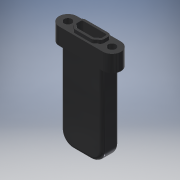
# Autodesk Inventor part: hdmi-panel-mount
Saved by Autodesk Inventor 2017 (Build 210142000, 142)
## iProperties
Created: 2020-10-05
Part Number: hdmi-panel-mount
Material: Generic
Document SubType Name: Modeling
Designer: Joe Ferner
Density: 1 g/cm^3
Appearance: Default
Author: Joe Ferner
Autodesk Inventor part; units mm, degrees
ref_plane "YZ Plane" through (0, 0, 0) normal (1, 0, 0) x (0, 1, 0)
ref_plane "XZ Plane" through (0, 0, 0) normal (0, 1, 0) x (-1, 0, 0)
ref_plane "XY Plane" through (0, 0, 0) normal (0, 0, 1) x (1, 0, 0)
sketch "Sketch1" plane through (0, 0, 0) normal (0, 0, 1) x (1, 0, 0)
  line L0 (0, 0) -> (26.3, 0)
  line L1 (26.3, 10.7) -> (0, 10.7)
  arc A0 (0, 10.7) -> (0, 0) centre (0, 5.35) ccw
  arc A1 (26.3, 0) -> (26.3, 10.7) centre (26.3, 5.35) ccw
  circle A2 centre (0, 5.35) radius 1.25
  circle A3 centre (26.3, 5.35) radius 1.25
  dimension "d0" = 26.3
  dimension "d1" = 10.7
  dimension "d2" = 2.5
  constraints: 4 centre point, 4 end point, 4 point on circle, 4 tangent, 2 coincident, 1 equal radius, 1 horizontal, 1 parallel
  measures "d0" distance of L0.start L0.end
  measures "d1" distance between parallel lines of L1 L0
  measures "d2" diameter of A2
extrude "Extrusion1" add sketch "Sketch1" against normal blind 10
sketch "Sketch2" plane through (0, 0, 0) normal (0, 0, 1) x (1, 0, 0)
  line L0 (0, 0) -> (26.3, 0) projected
  arc A0 (0, 10.7) -> (0, 0) centre (0, 5.35) ccw projected
  line L1 (6.9455, 3.7725) -> (7.7604, 2.8465)
  line L2 (8.361, 2.575) -> (17.939, 2.575)
  line L3 (18.5396, 2.8465) -> (19.3545, 3.7725)
  line L4 (19.6057, 3.9348) -> (20.0852, 4.0824)
  line L5 (20.65, 4.847) -> (20.65, 7.325)
  line L6 (19.85, 8.125) -> (6.45, 8.125)
  line L7 (5.65, 7.325) -> (5.65, 4.847)
  line L8 (6.2148, 4.0824) -> (6.6943, 3.9348)
  line L9 (26.3, 10.7) -> (0, 10.7) projected
  arc A1 (6.45, 8.125) -> (5.65, 7.325) centre (6.45, 7.325) ccw
  arc A2 (20.65, 7.325) -> (19.85, 8.125) centre (19.85, 7.325) ccw
  arc A3 (5.65, 4.847) -> (6.2148, 4.0824) centre (6.45, 4.847) ccw
  arc A4 (20.0852, 4.0824) -> (20.65, 4.847) centre (19.85, 4.847) ccw
  arc A5 (6.9455, 3.7725) -> (6.6943, 3.9348) centre (6.5326, 3.4092) ccw
  arc A6 (19.6057, 3.9348) -> (19.3545, 3.7725) centre (19.7674, 3.4092) ccw
  arc A7 (7.7604, 2.8465) -> (8.361, 2.575) centre (8.361, 3.375) ccw
  arc A8 (17.939, 2.575) -> (18.5396, 2.8465) centre (17.939, 3.375) ccw
  line L10 (6.45, 9.4895) -> (19.85, 9.4895)
  arc A9 (22.0145, 7.325) -> (19.85, 9.4895) centre (19.85, 7.325) ccw
  line L11 (22.0145, 7.325) -> (22.0145, 4.847)
  arc A10 (20.4865, 2.7782) -> (22.0145, 4.847) centre (19.85, 4.847) ccw
  line L12 (20.4865, 2.7782) -> (20.2268, 2.6983)
  line L13 (20.2268, 2.6983) -> (19.5639, 1.945)
  arc A11 (17.939, 1.2105) -> (19.5639, 1.945) centre (17.939, 3.375) ccw
  line L14 (17.939, 1.2105) -> (8.361, 1.2105)
  arc A12 (6.7361, 1.945) -> (8.361, 1.2105) centre (8.361, 3.375) ccw
  line L15 (6.7361, 1.945) -> (6.0732, 2.6983)
  line L16 (6.0732, 2.6983) -> (5.8135, 2.7782)
  arc A13 (4.2855, 4.847) -> (5.8135, 2.7782) centre (6.45, 4.847) ccw
  line L17 (4.2855, 4.847) -> (4.2855, 7.325)
  arc A14 (6.45, 9.4895) -> (4.2855, 7.325) centre (6.45, 7.325) ccw
  point P0 (6.8428, 3.8892)
  point P1 (7.9994, 2.575)
  point P2 (18.3006, 2.575)
  point P3 (19.4572, 3.8892)
  point P4 (20.65, 4.2561)
  point P5 (20.65, 8.125)
  point P6 (5.65, 8.125)
  point P7 (5.65, 4.2561)
  dimension "d25" = 15
  dimension "d26" = 5.55
  dimension "d27" = 5.65
  dimension "d28" = 2.575
  dimension "d29" = 0.8
  dimension "d30" = 0.8
  dimension "d32" = 107.1
  dimension "d34" = 107.1
  dimension "d35" = 41.35
  dimension "d36" = 41.35
  dimension "d37" = 0.55
  dimension "d38" = 0.8
  dimension "d39" = 2.711
  dimension "d40" = 2.711
  dimension "d42" = 2.478
  dimension "d43" = 2.478
  dimension "d44" = 1.3645
  constraints: 32 end point, 28 point on circle, 16 point on line, 16 tangent, 14 centre point, 4 equal radius, 4 parallel, 2 perpendicular, 13 other
  measures "d25" distance between parallel lines of L5 L7
  measures "d26" distance between parallel lines of L6 L2
  measures "d27" distance from line of A0.centre L7
  measures "d28" distance between parallel lines of L9 L6
  measures "d29" radius of A1
  measures "d30" radius of A3
  measures "d32" angle of L8 L7
  measures "d34" angle of L4 L5
  measures "d35" angle of L1 L7
  measures "d36" angle of L5 L3
  measures "d37" radius of A5
  measures "d38" radius of A7
  measures "d39" distance from line of L2.start L7
  measures "d40" distance from line of L2.end L5
  measures "d42" distance of L7.start L7.end
  measures "d43" distance of L5.start L5.end
  measures "d44" distance between parallel lines of L2 L14
extrude "Extrusion4" add sketch "Sketch2" along normal blind 2 contours A5 L8 A3 L7 A1 L6 A2 L5 A4 L4 A6 L3 A8 L2 A7 L1 | L10 A9 L11 A10 L12 L13 A11 L14 A12 L15 L16 A13 L17 A14
extrude "Extrusion5" cut sketch "Sketch2" against normal blind 4 and the other way blind 2 contours A5 L8 A3 L7 A1 L6 A2 L5 A4 L4 A6 L3 A8 L2 A7 L1
sketch "Sketch3" plane through (0, 0, -10) normal (0, 0, -1) x (-1, 0, 0)
  line L0 (-23.4, 0) -> (-2.9, 0)
  line L1 (-2.9, 0) -> (-2.9, 10.7)
  line L2 (-2.9, 10.7) -> (-23.4, 10.7)
  line L3 (-23.4, 10.7) -> (-23.4, 0)
  line L4 (0, 10.7) -> (-26.3, 10.7) projected
  arc A0 (-26.3, 10.7) -> (-26.3, 0) centre (-26.3, 5.35) ccw projected
  line L5 (-26.3, 0) -> (0, 0) projected
  dimension "d47" = 20.5
  dimension "d51" = 2.9
  constraints: 8 end point, 2 collinear, 2 parallel, 1 horizontal, 1 perpendicular
  measures "d47" distance of L0.start L0.end
  measures "d51" distance from line of A0.centre L3
extrude "Extrusion6" add sketch "Sketch3" along normal blind 24 contours L3 L2 L1 L0
sketch "Sketch4" plane through (2.9, 10.7, -10) normal (0, 1, 0) x (-1, 0, 0)
  line L0 (-20.5, 0) -> (-20.5, -24) projected
  line L1 (-20.5, -24) -> (0, -24) projected
  arc A0 (-20.5, -21) -> (-17.5, -24) centre (-17.5, -21) ccw
  arc A1 (-3, -24) -> (0, -21) centre (-3, -21) ccw
  line L2 (-20.5, -21) -> (-20.5, -24)
  line L3 (-20.5, -24) -> (-17.5, -24)
  line L4 (-3, -24) -> (0, -24)
  line L5 (0, -24) -> (0, -21)
  line L6 (0, 0) -> (0, -24) projected
  point P0 (2.9, 10)
  dimension "d58" = 3
  dimension "d59" = 3
  dimension "d63" = 3
  dimension "d64" = 3
  dimension "d65" = 3
  dimension "d66" = 3
  constraints: 8 end point, 4 collinear, 4 point on circle, 3 point on line, 2 centre point, 1 vertical alignment
  measures "d58" radius of A0
  measures "d59" radius of A1
  measures "d63" distance from line of L2.start L1
  measures "d64" distance of L0.end L3.end
  measures "d65" distance of L1.end L4.start
  measures "d66" distance of L5.end L1.end
extrude "Extrusion7" cut sketch "Sketch4" against normal through all
fillet "Fillet1" radius 1 10 edges at (22.5213, 10.7, -33.1213) (13.15, 10.7, -34) (3.7787, 10.7, -33.1213) (2.9, 10.7, -20.5) (23.4, 10.7, -20.5) (22.5213, 0, -33.1213) (13.15, 0, -34) (3.7787, 0, -33.1213) (2.9, 0, -20.5) (23.4, 0, -20.5)
sketch "Sketch5" plane through (0, 0, -34) normal (0, 0, -1) x (-1, 0, 0)
  circle A0 centre (-13.15, 5.35) radius 4.7
  line L0 (-5.9, 10.7) -> (-20.4, 10.7) projected
  line L1 (-23.4, 1) -> (-23.4, 9.7) projected
  point P0 (0, 0)
  dimension "d67" = 9.4
  dimension "d68" = 5.35
  dimension "d69" = 10.25
  constraints: 1 centre point
  measures "d67" diameter of A0
  measures "d68" distance from line of L0 A0.centre
  measures "d69" distance from line of L1 A0.centre
extrude "Extrusion8" add sketch "Sketch5" along normal blind 8.8
equation "\"d27\" = -0.5 * d25 + 0.5 * d0"
equation "\"d28\" = -0.5 * d26 + 0.5 * d1"
equation "\"d34\" = d32"
equation "\"d36\" = d35"
equation "\"d40\" = d39"
equation "\"d43\" = d42"
equation "\"d51\" = -0.5 * d47 + 0.5 * d0"
equation "\"d58\" = d54"
equation "\"d59\" = d54"
equation "\"d63\" = d54"
equation "\"d64\" = d54"
equation "\"d65\" = d54"
equation "\"d66\" = d54"
equation "\"d68\" = 0.5 * d1"
equation "\"d69\" = 0.5 * d47"
equation "\"d54\" = 3"
body "Solid1"
